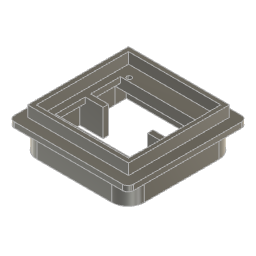
FIRE EXT RECESS v5 (Autodesk Fusion 360 design; units mm, degrees)
Autodesk Fusion 360 part; units mm, degrees
sketch "Sketch1" plane through (0, 0, 0) normal (0, 0, 1) x (1, 0, 0)
  line L0 (9.9, 9.9) -> (-9.9, 9.9)
  line L1 (-9.9, 9.9) -> (-9.9, -9.9)
  line L2 (-9.9, -9.9) -> (9.9, -9.9)
  line L3 (9.9, -9.9) -> (9.9, 9.9)
  line L4 (9.9, 9.9) -> (-9.9, -9.9) construction
  line L5 (-9.9, 9.9) -> (9.9, -9.9) construction
  line L6 (11, -11) -> (-11, -11)
  line L7 (-11, -11) -> (-11, 11)
  line L8 (-11, 11) -> (11, 11)
  line L9 (11, 11) -> (11, -11)
  line L10 (11, -11) -> (-11, 11) construction
  line L11 (-11, -11) -> (11, 11) construction
  line L12 (8.9, -8.9) -> (-8.9, -8.9)
  line L13 (-8.9, -8.9) -> (-8.9, 8.9)
  line L14 (-8.9, 8.9) -> (8.9, 8.9)
  line L15 (8.9, 8.9) -> (8.9, -8.9)
  line L16 (8.9, -8.9) -> (-8.9, 8.9) construction
  line L17 (-8.9, -8.9) -> (8.9, 8.9) construction
  line L18 (8.4, -6) -> (-8.4, -6)
  line L19 (-8.4, -6) -> (-8.4, 6)
  line L20 (-8.4, 6) -> (8.4, 6)
  line L21 (8.4, 6) -> (8.4, -6)
  line L22 (8.4, -6) -> (-8.4, 6) construction
  line L23 (-8.4, -6) -> (8.4, 6) construction
  line L24 (8.0957, 8.0957) -> (-8.0957, 8.0957)
  line L25 (-8.0957, 8.0957) -> (-8.0957, -8.0957)
  line L26 (-8.0957, -8.0957) -> (8.0957, -8.0957)
  line L27 (8.0957, -8.0957) -> (8.0957, 8.0957)
  line L28 (8.0957, 8.0957) -> (-8.0957, -8.0957) construction
  line L29 (-8.0957, 8.0957) -> (8.0957, -8.0957) construction
  line L30 (8.9, -0.5) -> (-8.9, -0.5)
  line L31 (-8.9, -0.5) -> (-8.9, 0.5)
  line L32 (-8.9, 0.5) -> (8.9, 0.5)
  line L33 (8.9, 0.5) -> (8.9, -0.5)
  line L34 (8.9, -0.5) -> (-8.9, 0.5) construction
  line L35 (-8.9, -0.5) -> (8.9, 0.5) construction
  dimension "d1" = 19.8
  dimension "d2" = 19.8
  dimension "d3" = 22
  dimension "d4" = 22
  dimension "d5" = 17.8
  dimension "d6" = 17.8
  dimension "d7" = 16.8
  dimension "d8" = 12
  dimension "d53" = 1
  constraint horizontal L0
  constraint perpendicular L0 L1
  constraint parallel L0 L2
  constraint parallel L1 L3
  constraint coincident L4 origin
  constraint coincident L5 origin
  constraint horizontal L6
  constraint perpendicular L6 L7
  constraint parallel L6 L8
  constraint parallel L7 L9
  constraint coincident L10 origin
  constraint coincident L11 origin
  constraint horizontal L12
  constraint perpendicular L12 L13
  constraint parallel L12 L14
  constraint parallel L13 L15
  constraint coincident L16 origin
  constraint coincident L17 origin
  constraint horizontal L18
  constraint perpendicular L18 L19
  constraint parallel L18 L20
  constraint parallel L19 L21
  constraint coincident L22 origin
  constraint coincident L23 origin
  constraint horizontal L24
  constraint perpendicular L24 L25
  constraint parallel L24 L26
  constraint parallel L25 L27
  constraint coincident L11 L24.start
  constraint coincident L28 origin
  constraint coincident L29 origin
  constraint horizontal L30
  constraint perpendicular L30 L31
  constraint parallel L30 L32
  constraint parallel L31 L33
  constraint coincident L34 origin
  constraint coincident L35 origin
  measures "d1" distance of L1.end L2.end
  measures "d2" distance of L0.end L1.end
  measures "d3" distance of L7.end L8.end
  measures "d4" distance of L6.end L7.end
  measures "d5" distance of L13.end L14.end
  measures "d6" distance of L12.end L13.end
  measures "d7" distance of L19.end L20.end
  measures "d8" distance of L18.end L19.end
  measures "d53" distance of L30.end L31.end
extrude "Extrude1" add sketch "Sketch1" along normal blind 1 contours L12 L13 L15 L18 L19 L21 L25 L26 L27 L30 | L15 L21 L30 L32 L33 | L13 L19 L30 L31 L32 | L13 L14 L15 L19 L20 L21 L24 L25 L27 L32 | L18 L25 L26 L27 | L20 L24 L25 L27
extrude "Extrude2" add sketch "Sketch1" along normal blind 4 contours L0 L1 L2 L3
extrude "Extrude3" add sketch "Sketch1" along normal blind 5 contours L6 L7 L8 L9
extrude "Extrude4" cut sketch "Sketch1" along normal blind 4 contours L6 L7 L8 L9
extrude "Extrude5" add 1 faces at (-9.5667, -2.9667, 4) along direction (0, 0, 1) blind 1
fillet "Fillet1" radius 3 1 edges at (9.9, -9.9, 2)
fillet "Fillet2" radius 3 1 edges at (-9.9, -9.9, 2)
fillet "Fillet3" radius 3 2 edges at (-9.9, 9.9, 2) (9.9, 9.9, 2)
fillet "Fillet4" radius 1 4 edges at (-11, -11, 4.5) (-11, 11, 4.5) (11, -11, 4.5) (11, 11, 4.5)
extrude "Extrude6" add 1 faces at (-2.8, -7.9333, 1) along direction (0, 0, 1) blind 5
extrude "Extrude7" cut sketch "Sketch1" along normal blind 3 contours L18 L25 L26 L27 | L20 L24 L25 L27
extrude "Extrude8" cut 1 faces at (-8.0957, 7.3972, 1) along direction (-1, 0, 0) blind 0.304
extrude "Extrude9" cut 1 faces at (8.0957, 6.6986, 1) along direction (1, 0, 0) blind 0.304
extrude "Extrude10" cut 1 faces at (8.0957, -7.3972, 1) along direction (1, 0, 0) blind 0.304
extrude "Extrude11" cut 1 faces at (-8.0957, -6.6986, 1) along direction (-1, 0, 0) blind 0.304
sketch "Sketch2" plane through (8.4, 0, 0) normal (-1, 0, 0) x (0, -1, 0)
  line L0 (-6, 0) -> (6, 0)
  line L1 (6, 0) -> (6, 6)
  line L2 (6, 6) -> (-6, 6)
  line L3 (-6, 6) -> (-6, 0)
  line L4 (-6, 6) -> (6, 6)
  line L5 (6, 6) -> (6, 4.0166)
  line L6 (6, 4.0166) -> (-6, 4.0166)
  line L7 (-6, 4.0166) -> (-6, 6)
  constraint horizontal L4
  constraint vertical L5
  constraint horizontal L6
  constraint vertical L7
  constraint coincident L1 L5.end
  constraint coincident L2.end L3.start
extrude "Extrude12" add sketch "Sketch2" along normal blind 1 contours L1 L2 L3 L4 L5 L6 L7
sketch "Sketch3" plane through (-8.4, 0, 0) normal (1, 0, 0) x (0, 1, 0)
  line L0 (-6, 0) -> (6, 0)
  line L1 (6, 0) -> (6, 6)
  line L2 (6, 6) -> (-6, 6)
  line L3 (-6, 6) -> (-6, 0)
  line L4 (-6, 6) -> (6, 6)
  line L5 (6, 6) -> (6, 3.9624)
  line L6 (6, 3.9624) -> (-6, 3.9624)
  line L7 (-6, 3.9624) -> (-6, 6)
  constraint horizontal L4
  constraint vertical L5
  constraint horizontal L6
  constraint vertical L7
  constraint coincident L1 L5.end
  constraint coincident L2.end L3.start
extrude "Extrude13" add sketch "Sketch3" along normal blind 1 contours L1 L2 L3 L4 L5 L6 L7
extrude "Extrude14" cut 1 faces at (-2.4667, 7.9333, 6) along direction (0, 0, -1) blind 2
extrude "Extrude15" add 1 faces at (-2.4667, 7.9333, 4) along direction (0, 0, 1) blind 1
sketch "TOP BUTTON GUIDE" plane through (0, 0, 5) normal (0, 0, 1) x (-1, 0, 0)
  line L0 (-8.4, 6) -> (7.4, 6)
  line L1 (7.4, 6) -> (7.4, -6)
  line L2 (7.4, -6) -> (-8.4, -6)
  line L3 (-8.4, -6) -> (-8.4, 6)
  arc A0 (-11, -10) -> (-10, -11) centre (-10, -10) ccw
  line L4 (-10, -11) -> (10, -11)
  arc A1 (10, -11) -> (11, -10) centre (10, -10) ccw
  line L5 (11, -10) -> (11, 10)
  arc A2 (11, 10) -> (10, 11) centre (10, 10) ccw
  line L6 (10, 11) -> (-10, 11)
  arc A3 (-10, 11) -> (-11, 10) centre (-10, 10) ccw
  line L7 (-11, 10) -> (-11, -10)
  line L8 (-8.35, 8.25) -> (8.35, 8.25)
  line L9 (8.35, 8.25) -> (8.35, -8.25)
  line L10 (8.35, -8.25) -> (-8.35, -8.25)
  line L11 (-8.35, -8.25) -> (-8.35, 8.25)
  line L12 (-8.35, 8.25) -> (8.35, -8.25) construction
  line L13 (8.35, 8.25) -> (-8.35, -8.25) construction
  line L14 (-9.15, 9.05) -> (9.15, 9.05)
  line L15 (9.15, 9.05) -> (9.15, -9.05)
  line L16 (9.15, -9.05) -> (-9.15, -9.05)
  line L17 (-9.15, -9.05) -> (-9.15, 9.05)
  line L18 (-9.15, 9.05) -> (9.15, -9.05) construction
  line L19 (9.15, 9.05) -> (-9.15, -9.05) construction
  dimension "d47" = 16.7
  dimension "d48" = 16.5
  dimension "d49" = 18.3
  dimension "d50" = 18.1
  constraint horizontal L8
  constraint perpendicular L8 L9
  constraint parallel L8 L10
  constraint parallel L9 L11
  constraint coincident L12 origin
  constraint coincident L13 origin
  constraint horizontal L14
  constraint perpendicular L14 L15
  constraint parallel L14 L16
  constraint parallel L15 L17
  constraint coincident L18 origin
  constraint coincident L19 origin
  measures "d47" distance of L9.end L10.end
  measures "d48" distance of L8.end L9.end
  measures "d49" distance of L15.end L16.end
  measures "d50" distance of L14.end L15.end
extrude "Extrude16" add sketch "TOP BUTTON GUIDE" along normal blind 2 contours L14 L15 L16 L17
extrude "Extrude17" add sketch "Sketch1" along normal blind 5 contours L21 L27 L30 L32 | L19 L25 L30 L32 | L25 L27 L30 L32
sketch "Sketch5" plane through (0, 0, 5) normal (0, 0, 1) x (-1, 0, 0)
  line L0 (7.4, -0.5) -> (7.4, -6)
  line L1 (7.4, -6) -> (-8.35, -6)
  line L2 (-8.35, -6) -> (-8.35, -8.25)
  line L3 (-8.35, -8.25) -> (8.35, -8.25)
  line L4 (8.35, -8.25) -> (8.35, 8.25)
  line L5 (8.35, 8.25) -> (-8.35, 8.25)
  line L6 (-8.35, 8.25) -> (-8.35, 6)
  line L7 (-8.35, 6) -> (7.4, 6)
  line L8 (7.4, 6) -> (7.4, 0.5)
  line L9 (7.4, 0.5) -> (-8.4, 0.5)
  line L10 (-8.4, 0.5) -> (-8.4, -0.5)
  line L11 (-8.4, -0.5) -> (7.4, -0.5)
  line L12 (-3.5, 1.3147) -> (3.5, 1.3147)
  line L13 (3.5, 1.3147) -> (3.5, -1.3147)
  line L14 (3.5, -1.3147) -> (-3.5, -1.3147)
  line L15 (-3.5, -1.3147) -> (-3.5, 1.3147)
  line L16 (-3.5, 1.3147) -> (3.5, -1.3147) construction
  line L17 (3.5, 1.3147) -> (-3.5, -1.3147) construction
  dimension "d56" = 7
  constraint horizontal L12
  constraint perpendicular L12 L13
  constraint parallel L12 L14
  constraint parallel L13 L15
  constraint coincident L16 origin
  constraint coincident L17 origin
  measures "d56" distance of L13.end L14.end
extrude "Extrude18" cut sketch "Sketch5" against normal blind 6 contours L9 L11 L13 L15
extrude "Extrude19" cut 1 faces at (-2.7833, 8.25, 5.6667) along direction (0, 1, 0) blind 0.5
extrude "Extrude20" add 1 faces at (-3.05, 9.05, 5.6667) along direction (0, 1, 0) blind 0.5
extrude "Extrude21" cut 1 faces at (-8.35, -2.5833, 5.6667) along direction (-1, 0, 0) blind 0.3
extrude "Extrude22" add 1 faces at (-9.15, 3.35, 5.6667) along direction (-1, 0, 0) blind 0.3
sketch "Sketch6" plane through (0, 0, 5) normal (0, 0, 1) x (-1, 0, 0)
  line L0 (3.5, 0.5) -> (3.5, -0.5)
  line L1 (3.5, -0.5) -> (7.4, -0.5)
  line L2 (7.4, -0.5) -> (7.4, -6)
  line L3 (7.4, -6) -> (-8.35, -6)
  line L4 (-8.35, -6) -> (-8.35, -8.75)
  line L5 (-8.35, -8.75) -> (8.65, -8.75)
  line L6 (8.65, -8.75) -> (8.65, 8.25)
  line L7 (8.65, 8.25) -> (-8.35, 8.25)
  line L8 (-8.35, 8.25) -> (-8.35, 6)
  line L9 (-8.35, 6) -> (7.4, 6)
  line L10 (7.4, 6) -> (7.4, 0.5)
  line L11 (7.4, 0.5) -> (3.5, 0.5)
  circle A0 centre (6.4473, -6.6661) radius 0.4424
extrude "Extrude23" cut sketch "Sketch6" against normal blind 2 contours A0
extrude "Extrude24" cut 1 faces at (-3.5, -0.1667, 3.3333) along direction (-1, 0, 0) blind 0.6
extrude "Extrude25" cut 1 faces at (3.5, 0.1667, 3.3333) along direction (1, 0, 0) blind 0.6
